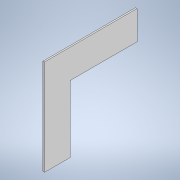
# Autodesk Inventor part: Side Part
Saved by Autodesk Inventor 2022.2 (Build 262287000, 287)
## iProperties
Created: 2022-02-23
Part Number: Side Part
Material: Generic
Document SubType Name: Modeling
Designer: PRASHANTH
Density: 1 g/cm^3
Appearance: Default
Author: PRASHANTH
Autodesk Inventor part; units mm, degrees
ref_plane "YZ Plane" through (0, 0, 0) normal (1, 0, 0) x (0, 1, 0)
ref_plane "XZ Plane" through (0, 0, 0) normal (0, 1, 0) x (-1, 0, 0)
ref_plane "XY Plane" through (0, 0, 0) normal (0, 0, 1) x (1, 0, 0)
sketch "Sketch1" plane through (0, 0, 0) normal (1, 0, 0) x (0, 1, 0)
  line L0 (157.5, -42.5) -> (157.5, 42.5)
  line L1 (157.5, 42.5) -> (-157.5, 42.5)
  line L2 (-157.5, 42.5) -> (-157.5, -42.5)
  line L3 (-157.5, -42.5) -> (62.5, -42.5)
  line L4 (62.5, -42.5) -> (62.5, -262.5)
  line L5 (62.5, -262.5) -> (157.5, -262.5)
  line L6 (157.5, -262.5) -> (157.5, -42.5)
  point P0 (0, 0)
  constraints: 14 end point, 1 horizontal, 1 parallel, 1 perpendicular, 1 vertical
extrude "Extrusion1" add sketch "Sketch1" along normal blind 5
body "Solid1"
